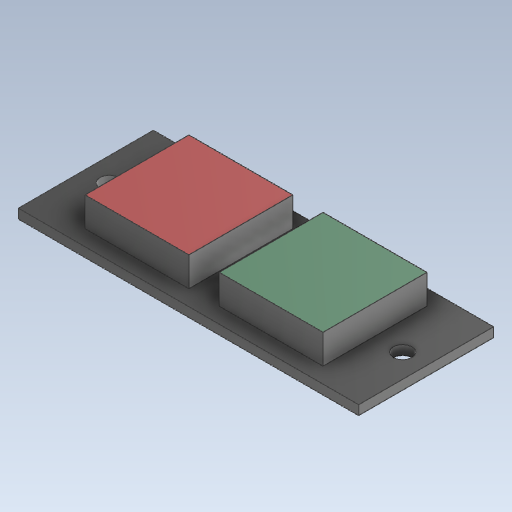
# Autodesk Inventor part: StartStopSwitch
Saved by Autodesk Inventor 2020.4 (Build 244396000, 396)
## iProperties
Created: 2022-03-29
Part Number: StartStopSwitch
Material: 一般
Document SubType Name: Modeling
Designer: Masato Kubotera
Density: 1 g/cm^3
Appearance: 滑らか - 黒
Author: Masato Kubotera
Autodesk Inventor part; units mm, degrees
ref_plane "YZ Plane" through (0, 0, 0) normal (1, 0, 0) x (0, 1, 0)
ref_plane "XZ Plane" through (0, 0, 0) normal (0, 1, 0) x (-1, 0, 0)
ref_plane "XY Plane" through (0, 0, 0) normal (0, 0, 1) x (1, 0, 0)
derived "Cockpit_top_frame.ipt"
sketch "スケッチ3" plane through (0, 0, -22.5) normal (0, 0, 1) x (1, 0, 0)
  line L0 (-84, -140) -> (-52.5, -140) construction
  line L1 (-52.5, -140) -> (-52.5, 5) construction
  line L2 (-52.5, 5) -> (-84, 5) construction
  line L3 (-84, 5) -> (-84, -140) construction
  line L4 (-84, -140) -> (-52.5, 5) construction
  line L5 (-52.5, -140) -> (-84, 5) construction
  line L6 (-72.25, 2.5) -> (-64.25, 2.5) construction
  line L7 (-64.25, 2.5) -> (-64.25, 0) construction
  line L8 (-64.25, 0) -> (-72.25, 0) construction
  line L9 (-72.25, 0) -> (-72.25, 2.5) construction
  line L10 (-72.25, 2.5) -> (-64.25, 0) construction
  line L11 (-64.25, 2.5) -> (-72.25, 0) construction
  line L12 (-79.05, 5) -> (-79.05, 0) construction
  line L13 (-79.05, 0) -> (-84, 0) construction
  arc A0 (-80.5349, 0) -> (-79.05, 1.4849) centre (-79.7925, 0.7425) ccw construction
  line L14 (-72.3, 2.55) -> (-64.2, 2.55) construction
  line L15 (-64.2, 2.55) -> (-64.2, -0.05) construction
  line L16 (-64.2, -0.05) -> (-72.3, -0.05) construction
  line L17 (-72.3, -0.05) -> (-72.3, 2.55) construction
  line L18 (-72.3, 2.55) -> (-64.2, -0.05) construction
  line L19 (-64.2, 2.55) -> (-72.3, -0.05) construction
  line L20 (-72.25, 1.25) -> (-64.25, 1.25) construction
  line L21 (-68.25, 2.5) -> (-68.25, 0) construction
  arc A1 (-70.8151, 2.55) -> (-72.3, 1.0651) centre (-71.5575, 1.8075) ccw construction
  arc A2 (-72.3, -0.05) -> (-70.2, -0.05) centre (-71.25, -0.05) ccw construction
  arc A3 (-64.2, 1.0651) -> (-65.6849, 2.55) centre (-64.9425, 1.8075) ccw construction
  arc A4 (-66.3, -0.05) -> (-64.2, -0.05) centre (-65.25, -0.05) ccw construction
  line L22 (-58.3142, -46.1342) -> (-78.1858, -66.0058) construction
  arc A5 (-60.3142, -66.0058) -> (-58.3142, -64.0058) centre (-60.3142, -64.0058) ccw construction
  line L23 (-68.25, -56.07) -> (-68.25, -78.93) construction
  arc A6 (-76.1858, -46.1342) -> (-78.1858, -48.1342) centre (-76.1858, -48.1342) ccw construction
  arc A7 (-58.3142, -48.1342) -> (-60.3142, -46.1342) centre (-60.3142, -48.1342) ccw construction
  line L24 (-76.1858, -66.0058) -> (-60.3142, -66.0058) construction
  line L25 (-58.9, -65.42) -> (-77.6, -65.42) construction
  line L26 (-58.3142, -64.0058) -> (-58.3142, -48.1342) construction
  line L27 (-78.1858, -48.1342) -> (-78.1858, -64.0058) construction
  line L28 (-77.6, -65.42) -> (-77.6, -46.72) construction
  line L29 (-77.6, -46.72) -> (-58.9, -46.72) construction
  line L30 (-77.6, -65.42) -> (-58.9, -46.72) construction
  line L31 (-58.9, -65.42) -> (-77.6, -46.72) construction
  line L32 (-58.9, -46.72) -> (-58.9, -65.42) construction
  line L33 (-78.1858, -46.1342) -> (-58.3142, -66.0058) construction
  arc A8 (-78.1858, -64.0058) -> (-76.1858, -66.0058) centre (-76.1858, -64.0058) ccw construction
  line L34 (-60.3142, -46.1342) -> (-76.1858, -46.1342) construction
  line L35 (-84, -67.5) -> (-52.5, -67.5) construction
  circle A9 centre (-75.625, 2.5) radius 1.6 construction
  circle A10 centre (-60.875, 2.5) radius 1.6 construction
  line L36 (-79.75, -96.5) -> (-56.75, -96.5)
  line L37 (-56.75, -96.5) -> (-56.75, -38.5)
  line L38 (-56.75, -38.5) -> (-79.75, -38.5)
  line L39 (-79.75, -38.5) -> (-79.75, -96.5)
  line L40 (-79.75, -96.5) -> (-56.75, -38.5) construction
  line L41 (-56.75, -96.5) -> (-79.75, -38.5) construction
  line L42 (-77.1, -47.22) -> (-59.4, -47.22)
  line L43 (-59.4, -47.22) -> (-59.4, -64.92)
  line L44 (-59.4, -64.92) -> (-77.1, -64.92)
  line L45 (-77.1, -64.92) -> (-77.1, -47.22)
  line L46 (-77.1, -47.22) -> (-59.4, -64.92) construction
  line L47 (-59.4, -47.22) -> (-77.1, -64.92) construction
  circle A11 centre (-68.25, -42.5) radius 1.6
  circle A12 centre (-68.25, -42.5) radius 2 construction
  line L48 (-59.4, -70.08) -> (-77.1, -70.08)
  line L49 (-59.4, -87.78) -> (-59.4, -70.08)
  line L50 (-77.1, -87.78) -> (-59.4, -87.78)
  line L51 (-77.1, -70.08) -> (-77.1, -87.78)
  circle A13 centre (-68.25, -92.5) radius 2 construction
  circle A14 centre (-68.25, -92.5) radius 1.6
  circle A15 centre (-68.25, -42.5) radius 3.5 construction
  point P0 (0, 0)
  point P1 (-68.25, -67.5)
  point P2 (-52.5, 0)
  point P3 (-68.25, 1.25)
  point P4 (-79, 0)
  point P5 (-79, 0)
  point P6 (-79, 0)
  point P7 (-68.25, -67.5)
  point P8 (-68.25, -67.5)
  point P9 (-68.25, -67.5)
  point P10 (-75.625, 0)
  point P11 (-75.625, 0)
  point P12 (-60.875, 0)
  point P13 (-60.875, 0)
  point P14 (-60.875, 0)
  point P15 (-68.25, -67.5)
extrude "押し出し1" add sketch "スケッチ3" against normal blind 1.6 contours L39 L38 L37 L36 | L42 L43 L44 L45 | L49 L50 L51 L48
extrude "押し出し2" add sketch "スケッチ3" along normal blind 5 contours L42 L43 L44 L45 | L49 L50 L51 L48
